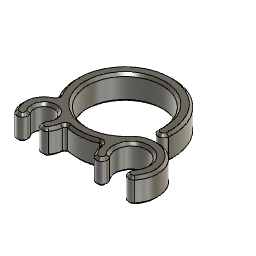
CableClipDual (Autodesk Fusion 360 design; units mm, degrees)
Autodesk Fusion 360 part; units mm, degrees
sketch "Sketch1" plane through (0, 0, 0) normal (0, 0, 1) x (1, 0, 0)
  circle A0 centre (0, 0) radius 7.5
  circle A1 centre (0, 0) radius 9.7
  circle A2 centre (9.6967, -8.3937) radius 3.125
  circle A3 centre (9.6967, -8.3937) radius 5.325
  circle A4 centre (-6.8033, -9.5187) radius 2
  line L0 (-19.1275, 0) -> (19.1275, 0) construction
  line L1 (0, 53.4087) -> (0, -53.4087) construction
  circle A5 centre (-6.8033, -9.5187) radius 4.2
  line L2 (-6.8033, 12) -> (-6.8033, -22) construction
  line L3 (9.6967, 12) -> (9.6967, -22) construction
  circle A6 centre (-9.3033, -11.3517) radius 1.1
  circle A7 centre (-4.3033, -11.3517) radius 1.1
  line L4 (-13.495, -11.3517) -> (0, -11.3517) construction
  circle A8 centre (6.4467, -11.0933) radius 1.1
  circle A9 centre (12.9467, -11.0933) radius 1.1
  line L5 (0, -11.0933) -> (16.5909, -11.0933) construction
  circle A10 centre (8.5673, -0.7495) radius 1.1
  line L6 (-19.1235, -13.7187) -> (19.1666, -13.7187) construction
  line L7 (0, 0) -> (8.5673, -0.7495) construction
  dimension "d5_1_1" = 15
  dimension "d6_1_1" = 2.2
  dimension "d7_1_1" = 6.25
  dimension "d9_1_1" = 2.2
  dimension "d11_1_1" = 2.2
  dimension "d12_1_1" = 4
  dimension "d15_1_1" = 2.2
  dimension "d16_1_1" = 2.2
  dimension "d17_1_1" = 2.2
  dimension "d18_1_1" = 2.2
  dimension "d19_1_1" = 5
  dimension "d20_1_1" = 6.5
  dimension "d23_1_1" = 2.2
  dimension "d27" = 95
  dimension "d29" = 16.5
  constraint coincident A0.centre A1.centre
  constraint concentric A0 A1
  constraint concentric A2 A3
  constraint horizontal L0
  constraint midpoint A0.centre L0
  constraint vertical L1
  constraint midpoint A0.centre L1
  constraint concentric A4 A5
  constraint vertical L2
  constraint vertical L3
  constraint coincident A4.centre L2
  constraint coincident A2.centre L3
  constraint tangent A0 A5
  constraint tangent A0 A3
  constraint tangent A4 A6
  constraint tangent A4 A7
  constraint coincident L1 L4.end
  constraint perpendicular L1 L4
  constraint coincident A7.centre L4
  constraint coincident A6.centre L4
  constraint tangent A2 A8
  constraint tangent A2 A9
  constraint coincident L1 L5.start
  constraint perpendicular L3 L5
  constraint coincident A9.centre L5
  constraint coincident A8.centre L5
  constraint tangent A0 A10
  constraint horizontal L6
  constraint tangent A5 L6
  constraint tangent A3 L6
  constraint coincident A10.centre L7.end
  measures "d5_1_1" diameter of A0
  measures "d6_1_1" distance of A0 A1
  measures "d7_1_1" diameter of A2
  measures "d9_1_1" distance of A2 A3
  measures "d11_1_1" distance of A4 A5
  measures "d12_1_1" diameter of A4
  measures "d15_1_1" diameter of A6
  measures "d16_1_1" diameter of A7
  measures "d17_1_1" diameter of A8
  measures "d18_1_1" diameter of A9
  measures "d19_1_1" distance of A6.centre A7.centre
  measures "d20_1_1" distance of A8.centre A9.centre
  measures "d23_1_1" diameter of A10
  measures "d27" angle of L1 L7
  measures "d29" distance of L2 L3
extrude "Extrude1" add sketch "Sketch1" along normal blind 5 contours A0 A1 A5 A10 | A0 A1 A3 A5 | A1 A5 | A10 | A1 A3 | A1 A4 A5 A7 | A1 A4 A5 A6 | A1 A2 A3 A9 | A1 A2 A3 A8 | A6 | A8 | A7 | A9
fillet "Fillet1" radius 0.5 3 edges at (-2.6069, -9.3431, 2.5) (4.3782, -8.6557, 2.5) (-7.9958, -5.4916, 2.5)
chamfer "Chamfer1" distance 0.5 angle 45 34 edges at (4.8641, -10.63, 0) (7.1496, -11.9395, 0) (9.6967, -5.2687, 0) (12.2439, -11.9395, 0) (13.1407, -4.3323, 0) (-6.9068, 2.9233, 0) (8.4714, -1.8454, 0) (-2.1754, 9.4529, 0) (-8.2731, -5.3898, 0) (-10.867, -8.4573, 0) (-8.6528, -12.2388, 0) (-6.8033, -7.5187, 0) (-4.9537, -12.2388, 0) (-2.8801, -11.0182, 0) (-2.4208, -9.5726, 0) (0.9139, -9.6568, 0) (4.1987, -8.9612, 0) (4.1987, -8.9612, 5) (4.8641, -10.63, 5) (7.1496, -11.9395, 5) (9.6967, -5.2687, 5) (12.2439, -11.9395, 5) (13.1407, -4.3323, 5) (-6.9068, 2.9233, 5) (8.4714, -1.8454, 5) (-2.1754, 9.4529, 5) (-8.2731, -5.3898, 5) (-10.867, -8.4573, 5) (-8.6528, -12.2388, 5) (-6.8033, -7.5187, 5) (-4.9537, -12.2388, 5) (-2.8801, -11.0182, 5) (-2.4208, -9.5726, 5) (0.9139, -9.6568, 5)
equation "d6_1_1 = ClipWall"
equation "d9_1_1 = ClipWall"
equation "d11_1_1 = ClipWall"
equation "d15_1_1 = ClipWall"
equation "d16_1_1 = ClipWall"
equation "d17_1_1 = ClipWall"
equation "d18_1_1 = ClipWall"
equation "d21_1_1 = Thickness"
equation "d23_1_1 = ClipWall"
equation "ClipWall = 2.2 mm"
equation "Thickness = 5 mm"
